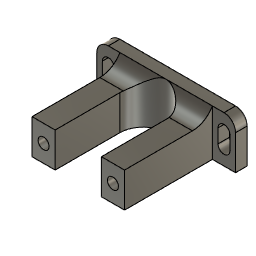
hemera_wiper (Autodesk Fusion 360 design; units mm, degrees)
Autodesk Fusion 360 part; units mm, degrees
sketch "Sketch1" plane through (0, 0, 0) normal (0, 1, 0) x (1, 0, 0)
  line L0 (-30, 10) -> (30, 10)
  line L1 (30, 10) -> (30, -10)
  line L2 (30, -10) -> (-30, -10)
  line L3 (-30, -10) -> (-30, 10)
  line L4 (-30, 10) -> (30, -10) construction
  line L5 (30, 10) -> (-30, -10) construction
  line L6 (20, 10) -> (-20, 10)
  line L7 (-20, 10) -> (-20, -10) construction
  line L8 (-20, -10) -> (20, -10)
  line L9 (20, -10) -> (20, 10) construction
  line L10 (20, 10) -> (-20, -10) construction
  line L11 (-20, 10) -> (20, -10) construction
  line L12 (-20, 10) -> (20, 10)
  line L13 (20, 10) -> (20, -5)
  line L14 (20, -5) -> (-20, -5)
  line L15 (-20, -5) -> (-20, 10)
  line L16 (0, -5) -> (0, 10) construction
  line L17 (10, -5) -> (-10, -5) construction
  line L18 (-10, -5) -> (-10, 10)
  line L19 (-10, 10) -> (10, 10) construction
  line L20 (10, 10) -> (10, -5)
  line L21 (10, -5) -> (-10, 10) construction
  line L22 (-10, -5) -> (10, 10) construction
  line L23 (-25, 10) -> (25, 10) construction
  line L24 (25, 10) -> (25, -10) construction
  line L25 (25, -10) -> (-25, -10) construction
  line L26 (-25, -10) -> (-25, 10) construction
  line L27 (-25, 10) -> (25, -10) construction
  line L28 (25, 10) -> (-25, -10) construction
  line L29 (25, -3) -> (-25, -3) construction
  line L30 (-25, -3) -> (-25, 3) construction
  line L31 (-25, 3) -> (25, 3) construction
  line L32 (25, 3) -> (25, -3) construction
  line L33 (25, -3) -> (-25, 3) construction
  line L34 (-25, -3) -> (25, 3) construction
  line L35 (27.6, -3) -> (27.6, 3)
  arc A0 (27.6, 3) -> (22.4, 3) centre (25, 3) ccw
  line L36 (22.4, 3) -> (22.4, -3)
  arc A1 (22.4, -3) -> (27.6, -3) centre (25, -3) ccw
  line L37 (25, -3) -> (25, 3) construction
  line L38 (-22.4, -3) -> (-22.4, 3)
  arc A2 (-22.4, 3) -> (-27.6, 3) centre (-25, 3) ccw
  line L39 (-27.6, 3) -> (-27.6, -3)
  arc A3 (-27.6, -3) -> (-22.4, -3) centre (-25, -3) ccw
  line L40 (-25, -3) -> (-25, 3) construction
  point P0 (0, 2.5)
  dimension "d1" = 60
  dimension "d2" = 20
  dimension "d3" = 40
  dimension "d4" = 15
  dimension "d5" = 20
  dimension "d10" = 50
  dimension "d11" = 6
  dimension "d12" = 5.2
  dimension "d13" = 5.2
  constraint horizontal L0
  constraint perpendicular L0 L1
  constraint parallel L0 L2
  constraint parallel L1 L3
  constraint coincident L4 origin
  constraint coincident L5 origin
  constraint horizontal L6
  constraint perpendicular L6 L7
  constraint parallel L6 L8
  constraint parallel L7 L9
  constraint coincident L10 origin
  constraint coincident L11 origin
  constraint horizontal L12
  constraint vertical L13
  constraint horizontal L14
  constraint vertical L15
  constraint midpoint L14 L16.start
  constraint midpoint L12 L16.end
  constraint horizontal L17
  constraint perpendicular L17 L18
  constraint parallel L17 L19
  constraint parallel L18 L20
  constraint coincident L21 P0
  constraint coincident L22 P0
  constraint midpoint L16 P0
  constraint horizontal L23
  constraint perpendicular L23 L24
  constraint parallel L23 L25
  constraint parallel L24 L26
  constraint coincident L27 origin
  constraint coincident L28 origin
  constraint horizontal L29
  constraint perpendicular L29 L30
  constraint parallel L29 L31
  constraint parallel L30 L32
  constraint coincident L33 origin
  constraint coincident L34 origin
  constraint tangent L35 A0
  constraint tangent A0 L36
  constraint parallel L35 L36
  constraint tangent L36 A1
  constraint tangent L35 A1
  constraint coincident L31.end L32.start
  constraint perpendicular L31 L37
  constraint coincident L29.start L32.end
  constraint tangent L38 A2
  constraint tangent A2 L39
  constraint parallel L38 L39
  constraint tangent L39 A3
  constraint tangent L38 A3
  constraint coincident L30.end L31.start
  constraint perpendicular L31 L40
  constraint coincident L29.end L30.start
  constraint coincident L26 L29.end
  measures "d1" distance of L1.end L2.end
  measures "d2" distance of L0.end L1.end
  measures "d3" distance of L7.end L8.end
  measures "d4" distance of L6.end L14.end
  measures "d5" distance of L18.end L19.end
  measures "d10" distance of L24.end L25.end
  measures "d11" distance of L29.end L30.end
  measures "d12" diameter of A0
  measures "d13" diameter of A2
extrude "Extrude1" add sketch "Sketch1" along normal blind 5
extrude "Extrude2" add sketch "Sketch1" against normal blind 38 contours L0 L6 L12 L14 L15 L18 | L0 L6 L12 L13 L14 L20
fillet "Fillet1" radius 10 4 edges at (-15, 0, 5) (-10, 0, -2.5) (15, 0, 5) (10, 0, -2.5)
fillet "Fillet2" radius 5 2 edges at (-30, 2.5, 10) (30, 2.5, 10)
hole "Hole1" at (-15, -38, -2.5) direction (0, 1, 0) diameter 4.8 depth 7.5 tip angle 180
mirror "Mirror1" about plane through (0, 0, 0) normal (1, 0, 0) of "Hole1"
